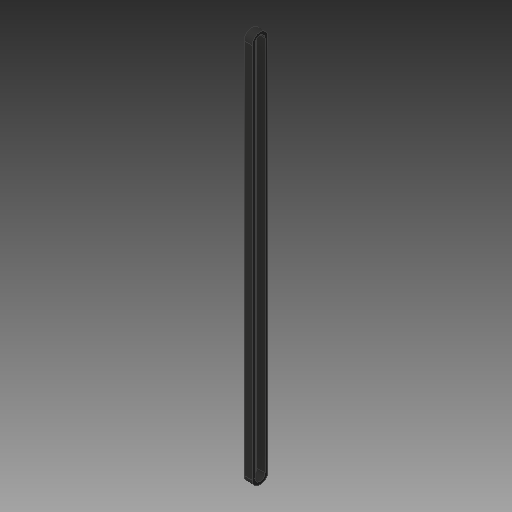
# Autodesk Inventor part: Long Belt
Saved by Autodesk Inventor 2019.4 (Build 234330000, 330)
## iProperties
Created: 2020-01-22
Part Number: Long Belt
Material: Rubber
Document SubType Name: Modeling
Designer: Mark
Mass: 108.23 g
Surface Area: 597.666 cm^2
Volume: 116.377 cm^3
Density: 0.93 g/cm^3
Appearance: Rubber - Black
Author: Mark
Autodesk Inventor part; units mm, degrees
ref_plane "YZ Plane" through (0, 0, 0) normal (1, 0, 0) x (0, 1, 0)
ref_plane "XZ Plane" through (0, 0, 0) normal (0, 1, 0) x (-1, 0, 0)
ref_plane "XY Plane" through (0, 0, 0) normal (0, 0, 1) x (1, 0, 0)
sketch "Sketch1" plane through (0, -135, 0) normal (1, 0, 0) x (0, 1, 0)
  arc A0 (0, 11.935) -> (0, -11.935) centre (0, 0) ccw
  arc A1 (700, -11.935) -> (700, 11.935) centre (700, 0) ccw
  line L0 (0, 11.935) -> (700, 11.935)
  line L1 (0, -11.935) -> (700, -11.935)
  line L2 (700, 0) -> (0, 0)
  line L3 (700, 9.305) -> (0, 9.305)
  arc A2 (0, 9.305) -> (0, -9.305) centre (0, 0) ccw
  line L4 (0, -9.305) -> (700, -9.305)
  arc A3 (700, -9.305) -> (700, 9.305) centre (700, 0) ccw
  line L5 (700, 14.565) -> (0, 14.565)
  arc A4 (0, 14.565) -> (0, -14.565) centre (0, 0) ccw
  line L6 (0, -14.565) -> (700, -14.565)
  arc A5 (700, -14.565) -> (700, 14.565) centre (700, 0) ccw
  dimension "d4" = 23.87
  dimension "d2" = 23.87
  dimension "d3" = 700
  dimension "d8" = 700
  dimension "d1" = 2.63
  dimension "d0" = 2.63
  constraints: 14 end point, 12 point on circle, 6 centre point, 4 tangent, 1 coincident, 6 other
  measures "d4" diameter of A0
  measures "d2" diameter of A1
  measures "d3" distance of L2.end L2.start
  measures "d8" distance of L2.start L2.end
  measures "d1" distance between parallel lines of L0 L3
  measures "d0" distance between parallel lines of L0 L5
extrude "Extrusion1" add sketch "Sketch1" along normal blind 15 contours L0 A1 L1 A0 | A5 L6 A4 L5
body "Solid1"
